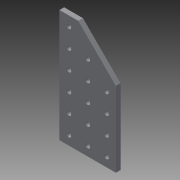
# Autodesk Inventor part: MAKERSLIDE_RISERS
Saved by Autodesk Inventor 2013 (Build 170138000, 138)
## iProperties
Created: 2013-06-20
Part Number: MAKERSLIDE_RISERS
Material: Generic
Document SubType Name: Modeling
Designer: Brett
Density: 1 g/cm^3
Author: Brett
Autodesk Inventor part; units mm, degrees
ref_plane "YZ Plane" through (0, 0, 0) normal (1, 0, 0) x (0, 1, 0)
ref_plane "XZ Plane" through (0, 0, 0) normal (0, 1, 0) x (-1, 0, 0)
ref_plane "XY Plane" through (0, 0, 0) normal (0, 0, 1) x (1, 0, 0)
sketch "Sketch2" plane through (0, 0, 0) normal (0, 0, 1) x (1, 0, 0)
  line L0 (-10, -10) -> (-10, 110)
  line L1 (-10, 110) -> (10, 110)
  line L2 (10, 110) -> (50, 70)
  line L3 (50, 70) -> (50, -10)
  line L4 (50, -10) -> (-10, -10)
  circle A0 centre (40, 0) radius 2.5
  circle A1 centre (40, 20) radius 2.5
  circle A2 centre (40, 40) radius 2.5
  circle A3 centre (40, 60) radius 2.5
  circle A4 centre (20, 80) radius 2.5
  circle A5 centre (20, 60) radius 2.5
  circle A6 centre (20, 40) radius 2.5
  circle A7 centre (20, 20) radius 2.5
  circle A8 centre (20, 0) radius 2.5
  circle A9 centre (0, 0) radius 2.5
  circle A10 centre (0, 20) radius 2.5
  circle A11 centre (0, 40) radius 2.5
  circle A12 centre (0, 60) radius 2.5
  circle A13 centre (0, 80) radius 2.5
  circle A14 centre (0, 100) radius 2.5
  constraints: 15 centre point, 14 equal radius, 10 end point, 2 perpendicular, 1 parallel
extrude "Extrusion1" add sketch "Sketch2" along normal blind 5
body "Solid1"
